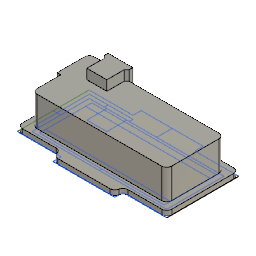
Emotibit_pour_moule (Autodesk Fusion 360 design; units mm, degrees)
Autodesk Fusion 360 part; units mm, degrees
sketch "Sketch1" plane through (0, 0, 0) normal (0, 0, 1) x (1, 0, 0)
  line L0 (-50, 18.3) -> (-50, -10.5)
  line L1 (-50, -10.5) -> (-32.4, -10.5)
  line L2 (-32.4, -10.5) -> (-32.4, -13.8)
  line L3 (-32.4, -13.8) -> (-7.6, -13.8)
  line L4 (-7.6, -13.8) -> (-7.6, -10.5)
  line L5 (-7.6, -10.5) -> (10, -10.5)
  line L6 (10, -10.5) -> (10, 18.3)
  line L7 (10, 18.3) -> (-7.6, 18.3)
  line L8 (-7.6, 18.3) -> (-7.6, 21.6)
  line L9 (-7.6, 21.6) -> (-32.4, 21.6)
  line L10 (-32.4, 21.6) -> (-32.4, 18.3)
  line L11 (-32.4, 18.3) -> (-50, 18.3)
  line L12 (-47, 15.4) -> (7, 15.4)
  line L13 (7, 15.4) -> (7, -7.6)
  line L14 (7, -7.6) -> (-47, -7.6)
  line L15 (-47, -7.6) -> (-47, 15.4)
  line L16 (-50, 3.9) -> (-47, 3.9)
  line L17 (-20, 15.4) -> (-20, 21.6)
  line L18 (-40, 15.4) -> (-40, 7.4)
  line L19 (-40, 7.4) -> (-32, 7.4)
  line L20 (-32, 7.4) -> (-32, 15.4)
  line L21 (-45, -6.6) -> (5, -6.6)
  line L22 (5, -6.6) -> (5, -4.1)
  line L23 (5, -4.1) -> (-45, -4.1)
  line L24 (-45, -4.1) -> (-45, -6.6)
  line L25 (-20, -6.6) -> (-20, -7.6)
  line L26 (-45, 14.4) -> (5, 14.4)
  line L27 (5, 14.4) -> (5, 11.9)
  line L28 (-45, 11.9) -> (-45, 14.4)
  line L29 (5, 11.9) -> (-45, 11.9)
  line L30 (-45, 11.9) -> (-45, -4.1)
  line L31 (5, 11.9) -> (5, -4.1)
  line L32 (-31, 15.4) -> (-31, 16.9)
  line L33 (-31, 16.9) -> (-48.5, 16.9)
  line L34 (-48.5, 16.9) -> (-48.5, -4.5956)
  line L35 (-48.5, -4.5956) -> (-47, -4.5956)
  line L36 (-41, 15.4) -> (-41, 16.9)
  dimension "d1" = 60
  dimension "d2" = 24.8
  dimension "d3" = 28.8
  dimension "d4" = 35.4
  dimension "d8" = 23
  dimension "d9" = 54
  dimension "d10" = 8
  dimension "d11" = 8
  dimension "d12" = 7
  dimension "d13" = 1
  dimension "d14" = 2.5
  dimension "d15" = 50
  dimension "d153" = 1.5
  dimension "d154" = 1.5
  dimension "d155" = 1
  dimension "d156" = 1
  measures "d1" distance of L0 L6
  measures "d2" distance of origin
  measures "d4" distance of L3 L9
  measures "d12" distance of L15 L18
  measures "d13" distance of L14 L21
  measures "d155" distance of L20 L32
  measures "d156" distance of L18 L36
extrude "Extrude2" add sketch "Sketch1" along normal blind 18 contours L12 L32 L33 L36 | L12 L18 L20 L26 | L18 L20 L26 L29 | L18 L19 L20 L29
extrude "Extrude3" add sketch "Sketch1" along normal blind 14 contours L12 L15 L16 L33 L34 L36 | L12 L14 L15 L18 L21 L24 L25 L26 L28 L30 | L12 L13 L14 L20 L21 L22 L25 L26 L27 L31 | L21 L22 L23 L24 | L18 L26 L28 L29 | L20 L26 L27 L29 | L18 L19 L20 L23 L29 L30 L31
extrude "Extrude5" add sketch "Sketch1" along normal blind 2 contours L0 L9 L10 L11 L12 L16 L17 L32 L33 L34 | L0 L1 L2 L3 L4 L5 L6 L7 L8 L9 L12 L13 L14 L15 L16 L17 L34 L35 | L12 L15 L16 L33 L34 L36 | L15 L16 L34 L35 | L12 L14 L15 L18 L21 L24 L25 L26 L28 L30 | L12 L32 L33 L36 | L12 L13 L14 L20 L21 L22 L25 L26 L27 L31 | L12 L18 L20 L26 | L18 L19 L20 L29 | L18 L19 L20 L23 L29 L30 L31
chamfer "Chamfer5" distance 1 angle 45 2 edges at (-40, 15.4, 16) (-32, 15.4, 16)
fillet "Fillet2" radius 2 12 edges at (-7.6, 18.3, 1) (-7.6, 21.6, 1) (-32.4, 21.6, 1) (-32.4, 18.3, 1) (-50, 18.3, 1) (-50, -10.5, 1) (-32.4, -10.5, 1) (-32.4, -13.8, 1) (-7.6, -10.5, 1) (-7.6, -13.8, 1) (10, -10.5, 1) (10, 18.3, 1)
fillet "Fillet26" radius 2 4 edges at (7, 15.4, 8) (7, -7.6, 8) (-47, -7.6, 8) (-48.5, 16.9, 8)
named bodies: "Emotibit"
